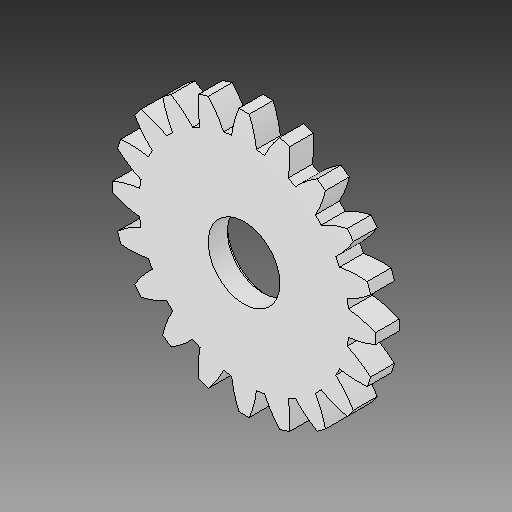
# Autodesk Inventor part: z20ギア(インベンター)
Saved by Autodesk Inventor 2019 (Build 230136000, 136)
## iProperties
Created: 2019-10-30
Part Number: z20ギア(インベンター)
Material: アセタール樹脂、白
Document SubType Name: Modeling
Designer: tanjihayato
Density: 1.425 g/cm^3
Appearance: 滑らか - 白
Mass: 6.45565 g
Surface Area: 34.3041 cm^2
Volume: 4.53028 cm^3
Author: tanjihayato
Autodesk Inventor part; units mm, degrees
ref_plane "YZ Plane" through (0, 0, 0) normal (1, 0, 0) x (0, 1, 0)
ref_plane "XZ Plane" through (0, 0, 0) normal (0, 1, 0) x (-1, 0, 0)
ref_plane "XY Plane" through (0, 0, 0) normal (0, 0, 1) x (1, 0, 0)
sketch "スケッチ1" plane through (0, 0, 0) normal (0, 0, 1) x (1, 0, 0)
  circle A0 centre (0, 0) radius 6
  circle A1 centre (0, 0) radius 6.8
  circle A2 centre (0, 0) radius 22
  dimension "d0" = 12
  dimension "d1" = 0.8
  dimension "d2" = 44
  constraints: 3 centre point, 2 coincident
  measures "d0" diameter of A0
  measures "d1" radial gap between concentric circles of A0 A1
  measures "d2" diameter of A2
extrude "押し出し1" add sketch "スケッチ1" along normal blind 4 contours A1 | A2
extrude "押し出し2" cut sketch "スケッチ1" along normal blind 0.8 contours A1
spur gear teeth "平歯車1" teeth 20 pitch diameter 40 tip diameter 44 root diameter 35.2 face width 4 trims to tip circle yes start plane through (0, 0, 0) normal (0, 0, -1) x (-1, 0, 0)
